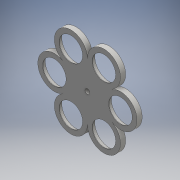
# Autodesk Inventor part: generator 12smaller
Saved by Autodesk Inventor 2016 (Build 200138000, 138)
## iProperties
Created: 2015-06-26
Part Number: generator 12smaller
Material: Generic
Document SubType Name: Modeling
Designer: KJardine
Density: 1 g/cm^3
Appearance: Default
Author: KJardine
Autodesk Inventor part; units mm, degrees
ref_plane "YZ Plane" through (0, 0, 0) normal (1, 0, 0) x (0, 1, 0)
ref_plane "XZ Plane" through (0, 0, 0) normal (0, 1, 0) x (-1, 0, 0)
ref_plane "XY Plane" through (0, 0, 0) normal (0, 0, 1) x (1, 0, 0)
sketch "Sketch1" plane through (0, 0, 0) normal (0, 1, 0) x (-1, 0, 0)
  circle A0 centre (0, 0) radius 55
  circle A1 centre (0, 0) radius 2.6
  dimension "d0" = 110
  dimension "d1" = 5.2
  constraints: 2 centre point, 2 coincident
  measures "d0" diameter of A0
  measures "d1" diameter of A1
extrude "Extrusion1" add sketch "Sketch1" along normal blind 5
sketch "Sketch2" plane through (0, 5, 0) normal (0, 1, 0) x (1, 0, 0)
  point P0 (0, 0)
sketch "Sketch4" plane through (0, 5, 0) normal (0, 1, 0) x (1, 0, 0)
  circle A0 centre (0, 0) radius 21.9076
  circle A1 centre (0, 0) radius 35
  circle A2 centre (-35, 0) radius 15.2
  circle A3 centre (-17.5, -30.3109) radius 15.2
  circle A4 centre (17.5, -30.3109) radius 15.2
  circle A5 centre (35, 0) radius 15.2
  circle A6 centre (17.5, 30.3109) radius 15.2
  circle A7 centre (-17.5, 30.3109) radius 15.2
  circle A8 centre (-21.9076, 0) radius 5.15
  circle A9 centre (-15.491, -15.491) radius 5.15
  circle A10 centre (0, -21.9076) radius 5.15
  circle A11 centre (15.491, -15.491) radius 5.15
  circle A12 centre (21.9076, 0) radius 5.15
  circle A13 centre (15.491, 15.491) radius 5.15
  circle A14 centre (0, 21.9076) radius 5.15
  circle A15 centre (-15.491, 15.491) radius 5.15
  dimension "d13" = 70
  dimension "d8" = 30.4
  dimension "d11" = 360
  dimension "d14" = 10.3
  dimension "d17" = 360
  constraints: 14 centre point, 2 coincident, 2 horizontal alignment, 34 other
  measures "d8" diameter of A2
  measures "d14" diameter of A8
extrude "Extrusion3" cut sketch "Sketch4" against normal blind 5 contours A0 A12 A5 | A0 A12 | A12 A5 A0 | A0 A5 A1 A12 | A0 A5 A12 | A5 A1 | A6 A13 A0 | A0 A13 A6 | A6 A0 A13 | A13 A0 A6 A14 A1 | A1 A6 | A4 A11 A0 | A0 A11 A4 | A4 A1 A10 A0 A11 | A11 A0 A4 | A4 A1 | A6 A14 | A7 A14 A0 A15 A1 | A1 A7 | A10 A4 | A3 A1 | A1 A3 A9 A0 A10 | A7 A14 | A10 A3 | A7 A15 A0 | A2 A0 A8 A1 | A1 A2 | A15 A0 A7 | A0 A9 A3 | A3 A0 A9 | A15 A7 A0 | A2 A8 A0 | A0 A3 A9 | A0 A8 A2 | A8 A2 A0 | A0 A8 picked at (11.9722, 17.0625) picked at (16.7139, 17.1312) picked at (8.2786, 19.0961) picked at (16.7139, -17.1312) picked at (11.9722, -17.0625) picked at (8.2786, -19.0961) picked at (-8.2786, 19.0961) picked at (-16.7226, 17.1255) picked at (-8.2786, -19.0961) picked at (-16.7226, -17.1255) picked at (-11.9722, 17.0625) picked at (-11.9722, -17.0625)
sketch "Sketch5" plane through (0, 5, 0) normal (0, 1, 0) x (1, 0, 0)
  point P0 (0, 0)
sketch "Sketch6" plane through (0, 0, 0) normal (0, -1, 0) x (1, 0, 0)
  circle A0 centre (0, 0) radius 55
  constraints: 1 centre point, 1 coincident
extrude "Extrusion4" add sketch "Sketch6" along normal blind 0.5
sketch "Sketch7" plane through (0, 5, 0) normal (0, 1, 0) x (1, 0, 0)
  circle A0 centre (-35, 0) radius 15.2 projected
  circle A1 centre (-35, 0) radius 12.5
  circle A2 centre (-17.5, -30.3109) radius 15.2 projected
  circle A3 centre (-17.5, -30.3109) radius 12.5
  circle A4 centre (17.5, -30.3109) radius 15.2 projected
  circle A5 centre (17.5, -30.3109) radius 12.5
  circle A6 centre (35, 0) radius 15.2 projected
  circle A7 centre (35, 0) radius 12.5
  circle A8 centre (17.5, 30.3109) radius 15.2 projected
  circle A9 centre (17.5, 30.3109) radius 12.5
  circle A10 centre (-17.5, 30.3109) radius 15.2 projected
  circle A11 centre (-17.5, 30.3109) radius 12.5
  point P0 (0, 0)
  dimension "d23" = 25
  dimension "d24" = 25
  dimension "d25" = 25
  dimension "d26" = 25
  dimension "d27" = 25
  dimension "d28" = 25
  constraints: 6 centre point, 6 coincident
  measures "d23" diameter of A1
  measures "d24" diameter of A3
  measures "d25" diameter of A5
  measures "d26" diameter of A7
  measures "d27" diameter of A9
  measures "d28" diameter of A11
extrude "Extrusion5" cut sketch "Sketch7" against normal blind 86.25 contours A1 | A3 | A5 | A7 | A9 | A11
sketch "Sketch8" plane through (0, 5, 0) normal (0, 1, 0) x (1, 0, 0)
  circle A0 centre (0, 0) radius 2.6
  constraints: 1 centre point, 1 coincident
extrude "Extrusion6" cut sketch "Sketch8" against normal blind 86.25
sketch "Sketch9" plane through (0, 5, 0) normal (0, 1, 0) x (1, 0, 0)
  circle A0 centre (17.5, 30.3109) radius 15.2 projected
  arc A1 (26.25, 15.1554) -> (0, 30.3109) centre (17.5, 30.3109) ccw
  circle A2 centre (35, 0) radius 15.2 projected
  arc A3 (26.25, -15.1554) -> (26.25, 15.1554) centre (35, 0) ccw
  circle A4 centre (17.5, -30.3109) radius 15.2 projected
  arc A5 (0, -30.3109) -> (26.25, -15.1554) centre (17.5, -30.3109) ccw
  circle A6 centre (-17.5, -30.3109) radius 15.2 projected
  arc A7 (-26.25, -15.1554) -> (0, -30.3109) centre (-17.5, -30.3109) ccw
  circle A8 centre (-35, 0) radius 15.2 projected
  arc A9 (-26.25, 15.1554) -> (-26.25, -15.1554) centre (-35, 0) ccw
  circle A10 centre (-17.5, 30.3109) radius 15.2 projected
  arc A11 (0, 30.3109) -> (-26.25, 15.1554) centre (-17.5, 30.3109) ccw
  circle A12 centre (0, 0) radius 2.6 projected
  circle A13 centre (0, 0) radius 65.8368
  dimension "d33" = 35
  dimension "d34" = 35
  dimension "d35" = 35
  dimension "d36" = 35
  dimension "d37" = 35
  dimension "d38" = 35
  dimension "d39" = 131.6736
  constraints: 12 point on circle, 7 centre point, 7 coincident
  measures "d33" diameter of A1
  measures "d34" diameter of A3
  measures "d35" diameter of A5
  measures "d36" diameter of A7
  measures "d37" diameter of A9
  measures "d38" diameter of A11
  measures "d39" diameter of A13
extrude "Extrusion7" cut sketch "Sketch9" against normal blind 86.25 contours A13
body "Solid1"
